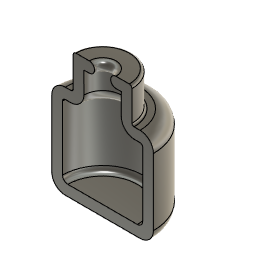
Sketch15_Final v4 (Autodesk Fusion 360 design; units mm, degrees)
Autodesk Fusion 360 part; units mm, degrees
sketch "Sketch1" plane through (0, 0, 0) normal (0, 1, 0) x (1, 0, 0)
  line L0 (0, 0) -> (-70, 0)
  line L1 (-95, -25) -> (-95, -150)
  line L2 (-70, -175) -> (-58.8, -175)
  line L3 (-55, -178.8) -> (-55, -235)
  line L4 (-50, -240) -> (-25, -240)
  line L5 (0, 0) -> (0, -20)
  line L6 (0, -20) -> (-65, -20)
  line L7 (-75, -30) -> (-74.9999, -149.9888)
  line L8 (-69.9886, -154.9887) -> (-59.8787, -154.966)
  line L9 (-34.8232, -179.7883) -> (-35, -219.9999)
  arc A0 (-95, -150) -> (-70, -175) centre (-70, -150) ccw
  arc A1 (-74.9999, -149.9888) -> (-69.9886, -154.9887) centre (-69.9999, -149.9888) ccw
  arc A2 (-55, -178.8) -> (-58.8, -175) centre (-58.8, -178.8) ccw
  arc A3 (-34.8232, -179.7883) -> (-59.8787, -154.966) centre (-59.8225, -179.966) ccw
  arc A4 (-65, -20) -> (-75, -30) centre (-65, -30) ccw
  arc A5 (-70, 0) -> (-95, -25) centre (-70, -25) ccw
  arc A6 (-55, -235) -> (-50, -240) centre (-50, -235) ccw
  line L10 (-35, -219.9999) -> (-25, -220)
  arc A7 (-25, -240) -> (-25, -220) centre (-25, -230) ccw
  point P0 (-95, 0)
  point P1 (-95, -175)
  point P2 (-55, -175)
  point P3 (-55, -240)
  point P4 (-95, -175)
  point P5 (-95, -175)
  point P6 (-74.9999, -155)
  point P7 (-35, -154.9101)
  point P8 (-55, -240)
  point P9 (-75, -20)
  point P10 (-95, 0)
  point P11 (-95, 0)
  dimension "d5" = 30
  dimension "d6" = 20
  dimension "d16" = 40
  dimension "d17" = 65
  dimension "d19" = 40
  dimension "d20" = 75
  dimension "d21" = 95
  dimension "d22" = 175
  dimension "d23" = 135
  dimension "d25" = 25
  dimension "d26" = 5
  dimension "d28" = 25
  constraint coincident L0.start L5.start
  constraint coincident P5 P4
  constraint coincident P11 P10
  constraint coincident P8 P3
  constraint coincident L8 P6
  constraint coincident L7 P6
  constraint coincident P2 L2
  measures "d5" distance of P8 L4.end
  measures "d6" distance of L0.start L5.end
  measures "d16" distance of P2 P5
  measures "d17" distance of P2 P8
  measures "d19" distance of P6 P7
  measures "d20" distance of L5.end P9
  measures "d21" distance of L0.start P11
  measures "d22" distance of P5 P11
  measures "d23" distance of P6 P9
  measures "d25" radius of A0
  measures "d26" radius of A1
  measures "d28" radius of A3
revolve "Revolve1" add sketch "Sketch1" angle 180 about axis through (0, 0, 1.75) along (0, 0, -1)
